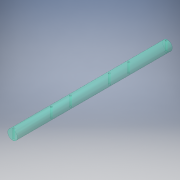
# Autodesk Inventor part: Straw
Saved by Autodesk Inventor 2016 (Build 200138000, 138)
## iProperties
Created: 2017-04-26
Part Number: Straw
Material: Generic
Document SubType Name: Modeling
Designer: wtse3759
Density: 1 g/cm^3
Appearance: Indoor Pool
Author: wtse3759
Autodesk Inventor part; units mm, degrees
ref_plane "YZ Plane" through (0, 0, 0) normal (1, 0, 0) x (0, 1, 0)
ref_plane "XZ Plane" through (0, 0, 0) normal (0, 1, 0) x (-1, 0, 0)
ref_plane "XY Plane" through (0, 0, 0) normal (0, 0, 1) x (1, 0, 0)
sketch "Sketch1" plane through (0, 0, 0) normal (0, 0, 1) x (1, 0, 0)
  circle A0 centre (0, 0) radius 6.35
  dimension "d0" = 12.7
  constraints: 1 centre point, 1 coincident
  measures "d0" diameter of A0
extrude "Extrusion1" add sketch "Sketch1" along normal blind 203.2
sketch "Sketch4" plane through (0, 0, 0) normal (0, 1, 0) x (-1, 0, 0)
  line L0 (0, 0) -> (0, 1.524)
  line L1 (6.35, 203.2) -> (-6.35, 203.2) projected
  line L2 (0, 203.2) -> (0, 201.676)
  circle A0 centre (0, 201.676) radius 1.27
  circle A1 centre (0, 1.524) radius 1.27
  dimension "d13" = 1.524
  dimension "d15" = 1.524
  dimension "d16" = 2.54
  dimension "d19" = 2.54
  constraints: 4 end point, 2 centre point, 2 coincident, 2 vertical, 1 midpoint
  measures "d13" distance of L0.start L0.end
  measures "d15" distance of L2.start L2.end
  measures "d16" diameter of A0
  measures "d19" diameter of A1
extrude "Extrusion4" cut sketch "Sketch4" along normal mid plane 15.24
sketch "Sketch8" plane through (0, 0, 0) normal (0, 1, 0) x (-1, 0, 0)
  line L0 (0, 0) -> (0, 50.8)
  circle A0 centre (0, 50.8) radius 1.27
  line L1 (0, 50.8) -> (0, 76.2)
  circle A1 centre (0, 76.2) radius 1.27
  line L2 (6.35, 203.2) -> (-6.35, 203.2) projected
  line L3 (0, 203.2) -> (0, 152.4)
  circle A2 centre (0, 152.4) radius 1.27
  line L4 (0, 152.4) -> (0, 127)
  circle A3 centre (0, 127) radius 1.27
  dimension "d50" = 50.8
  dimension "d51" = 2.54
  dimension "d58" = 25.4
  dimension "d59" = 2.54
  dimension "d60" = 50.8
  dimension "d61" = 2.54
  dimension "d62" = 25.4
  dimension "d63" = 2.54
  constraints: 8 end point, 4 centre point, 4 coincident, 3 vertical, 1 midpoint, 1 point on line
  measures "d50" distance of L0.start L0.end
  measures "d51" diameter of A0
  measures "d58" distance of L1.start L1.end
  measures "d59" diameter of A1
  measures "d60" distance of L3.start L3.end
  measures "d61" diameter of A2
  measures "d62" distance of L4.start L4.end
  measures "d63" diameter of A3
extrude "Extrusion10" cut sketch "Sketch8" along normal mid plane 25.4
body "Solid1"
